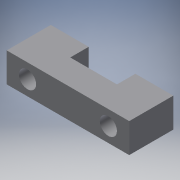
# Autodesk Inventor part: sensor bracket coupler
Saved by Autodesk Inventor 2017 SP1 (Build 210196100, 196)
## iProperties
Created: 2017-06-15
Part Number: sensor bracket coupler
Material: Generic
Document SubType Name: Modeling
Designer: RMcComber
Density: 1 g/cm^3
Appearance: Default
Author: RMcComber
Autodesk Inventor part; units mm, degrees
ref_plane "YZ Plane" through (0, 0, 0) normal (1, 0, 0) x (0, 1, 0)
ref_plane "XZ Plane" through (0, 0, 0) normal (0, 1, 0) x (-1, 0, 0)
ref_plane "XY Plane" through (0, 0, 0) normal (0, 0, 1) x (1, 0, 0)
sketch "Sketch1" plane through (0, 0, 0) normal (0, 0, 1) x (1, 0, 0)
  arc A0 (-4, 0) -> (4, 0) centre (0, 0) ccw
  line L0 (-4, 0) -> (-12.5, 0)
  line L1 (-12.5, 0) -> (-12.5, -10)
  line L2 (-12.5, -10) -> (12.5, -10)
  line L3 (12.5, -10) -> (12.5, 0)
  line L4 (12.5, 0) -> (4, 0)
  dimension "d0" = 4
  dimension "d1" = 10
  dimension "d2" = 25
  constraints: 10 end point, 3 collinear, 2 point on circle, 1 centre point, 1 coincident, 1 horizontal, 1 horizontal alignment, 1 parallel, 1 perpendicular, 1 vertical
  measures "d0" radius of A0
  measures "d1" distance of L0.end L1.end
  measures "d2" distance of L1.end L2.end
extrude "Extrusion1" add sketch "Sketch1" along normal blind 6
sketch "Sketch2" plane through (-12.5, 0, 0) normal (0, 1, 0) x (1, 0, 0)
  line L0 (0, 0) -> (8.5, 0) projected
  line L1 (8.5, -6) -> (0, -6) projected
  line L2 (16.5, 0) -> (25, 0) projected
  line L3 (16.5, 0) -> (16.5, -6) projected
  line L4 (25, -6) -> (16.5, -6) projected
  line L5 (25, 0) -> (25, -6) projected
  line L6 (4.25, 0) -> (4.25, -6) construction
  line L7 (20.75, 0) -> (20.75, -6) construction
  circle A0 centre (4.25, -3) radius 1.75
  circle A1 centre (20.75, -3) radius 1.75
  point P0 (12.5, 0)
  dimension "d5" = 3.5
  constraints: 6 midpoint, 4 end point, 2 centre point, 1 equal radius
  measures "d5" diameter of A0
extrude "Extrusion2" cut sketch "Sketch2" against normal through all contours A0 | A1
sketch "Sketch3" plane through (0, 0, 6) normal (0, 0, 1) x (1, 0, 0)
  line L0 (12.5, -10) -> (12.5, 0) projected
  line L1 (-12.5, 0) -> (12.5, 0)
  line L2 (12.5, 0) -> (12.5, -1)
  line L3 (12.5, -1) -> (-12.5, -1)
  line L4 (-12.5, -1) -> (-12.5, 0)
  dimension "d8" = 1
  constraints: 8 end point, 2 parallel, 1 horizontal, 1 perpendicular, 1 point on line
  measures "d8" distance of L3.end L1.start
extrude "Extrusion3" cut sketch "Sketch3" against normal through all
sketch "Sketch4" plane through (0, 0, 6) normal (0, 0, 1) x (1, 0, 0)
  line L0 (4.7625, -4.7625) -> (-4.7625, -4.7625)
  line L1 (-4.7625, -4.7625) -> (-4.7625, 4.7625)
  line L2 (-4.7625, 4.7625) -> (4.7625, 4.7625)
  line L3 (4.7625, 4.7625) -> (4.7625, -4.7625)
  line L4 (4.7625, -4.7625) -> (-4.7625, 4.7625) construction
  line L5 (-4.7625, -4.7625) -> (4.7625, 4.7625) construction
  point P0 (0, 0)
  dimension "d11" = 9.525
  constraints: 12 end point, 2 midpoint, 2 parallel, 2 perpendicular, 1 horizontal
  measures "d11" distance of L1.end L2.end
extrude "Extrusion4" cut sketch "Sketch4" against normal through all
body "Solid1"
